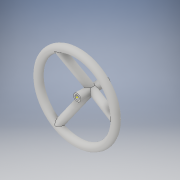
# Autodesk Inventor part: BaseThick
Saved by Autodesk Inventor 2019 (Build 230136000, 136)
## iProperties
Created: 2018-09-05
Part Number: BaseThick
Material: Generic
Document SubType Name: Modeling
Designer: s152529
Density: 1 g/cm^3
Appearance: Default
Author: s152529
Autodesk Inventor part; units mm, degrees
sketch "Sketch1" plane through (0, 0, 0) normal (0, 0, 1) x (1, 0, 0)
  circle A0 centre (0, 0) radius 52.5
  point P0 (52.5, 0)
  dimension "d0" = 105
  constraints: 2 horizontal alignment, 1 coincident, 2 other
ref_plane "Work Plane1" through (52.5, 0, 0) normal (0, 1, 0) x (-1, 0, 0)
sketch "Sketch2" plane through (52.5, 0, 0) normal (0, 1, 0) x (-1, 0, 0)
  circle A0 centre (0, 0) radius 5
  point P0 (52.5, 0)
  dimension "d1" = 10
  constraints: 1 centre point
  measures "d1" diameter of A0
sweep "Sweep1" add profiles "Sketch2" path "Sketch1"
sketch "Sketch3" plane through (52.5, 0, 0) normal (0, 1, 0) x (-1, 0, 0)
  point P0 (52.5, 0)
  point P1 (0, 0)
ref_plane "Work Plane2" through (0, 0, 0) normal (0, 1, 0) x (-1, 0, 0)
sketch "Sketch4" plane through (0, 0, 0) normal (0, 1, 0) x (-1, 0, 0)
  line L0 (0, -20) -> (-52.2148, 0)
  point P0 (0, 0)
  point P1 (-50.0579, -39.7962)
  dimension "d4" = 20
  constraints: 2 coincident, 2 end point
  measures "d4" distance of point (0, 0) L0.start
ref_plane "Work Plane3" through (0, 0, -20) normal (0.9338398, 0, 0.3576916) x (0, 1, 0)
sketch "Sketch5" plane through (0, 0, -20) normal (0.9338398, 0, 0.3576916) x (0, 1, 0)
  circle A0 centre (0, 0) radius 5
  point P0 (0, 18.6768)
  dimension "d5" = 10
  constraints: 1 centre point, 1 coincident
  measures "d5" diameter of A0
sweep "Sweep2" add profiles "Sketch5" path "Sketch4"
pattern_circular "Circular Pattern1" count 3 over 360 about axis through (0, 0, -10) along (0, 0, 1) of "Sweep2"
ref_plane "Work Plane4" through (0, 0, 0) normal (0, 0, 1) x (1, 0, 0)
sketch "Sketch6" plane through (0, 0, 0) normal (0, 0, 1) x (1, 0, 0)
  circle A0 centre (0, 0) radius 5
  dimension "d11" = 10
  constraints: 1 centre point, 1 coincident
  measures "d11" diameter of A0
extrude "Extrusion1" add sketch "Sketch6" against normal blind 40
ref_plane "Work Plane5" through (0, 5, 0) normal (0, 1, 0) x (-1, 0, 0)
sketch "Sketch7" plane through (0, 5, 0) normal (0, 1, 0) x (-1, 0, 0)
  line L0 (-5, -40) -> (5, -40) projected
  point P0 (0, 0)
  point P1 (0, -36)
  dimension "d28" = 4
  constraints: 1 vertical alignment
  measures "d28" distance from line of point (0, -36) L0
hole "Hole1" at (0, 5, -36) direction (0, -1, 0) diameter 5 end through all
sketch "Sketch8" plane through (0, 0, -40) normal (0, 0, -1) x (-1, 0, 0)
  point P0 (0, 0)
hole "Hole2" at (0, 0, -40) direction (0, 0, 1) diameter 6 end through all
body "Solid1"
